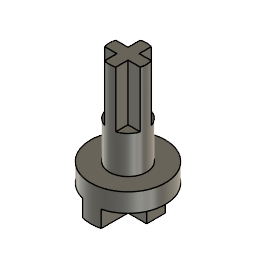
Potentiometer Axle Big (Autodesk Fusion 360 design; units mm, degrees)
part number: 2026-06-04-00-10-09-954
Autodesk Fusion 360 part; units mm, degrees
sketch "Sketch1" plane through (0, 0, 0) normal (0, 0, 1) x (1, 0, 0)
  circle A0 centre (0, 0) radius 1
  constraint coincident A0.centre origin
extrude "Extrude1" add sketch "Sketch1" along normal blind 0.5
sketch "Sketch2" plane through (0, 0, 0.5) normal (0, 0, 1) x (-1, 0, 0)
  circle A0 centre (0, 0) radius 1
  circle A1 centre (0, 0) radius 0.5
  constraint concentric A0 A1
extrude "Extrude2" add sketch "Sketch2" along normal blind 1 contours A1
sketch "Sketch3" plane through (0, 0, 1.5) normal (0, 0, 1) x (-1, 0, 0)
  circle A0 centre (0, 0) radius 0.5
  arc A1 (-0.1, -0.4899) -> (0.0992, -0.4901) centre (0, 0) ccw
  arc A2 (0.4899, -0.1) -> (0.4901, 0.0992) centre (0, 0) ccw
  arc A3 (0.1, 0.4899) -> (-0.1, 0.4899) centre (0, 0) ccw
  arc A4 (-0.4899, 0.1) -> (-0.4899, -0.1) centre (0, 0) ccw
  arc A5 (-0.15, -0.477) -> (0.15, -0.477) centre (0, 0) ccw
  arc A6 (-0.477, 0.15) -> (-0.477, -0.15) centre (0, 0) ccw
  arc A7 (0.477, -0.15) -> (0.477, 0.15) centre (0, 0) ccw
  arc A8 (0.15, 0.477) -> (-0.15, 0.477) centre (0, 0) ccw
  line L0 (-0.15, -0.15) -> (-0.15, -0.45)
  line L1 (-0.15, -0.45) -> (-0.15, -0.477)
  line L2 (-0.15, -0.15) -> (-0.477, -0.15)
  line L3 (0.15, -0.15) -> (0.15, -0.477)
  line L4 (0.15, -0.15) -> (0.477, -0.15)
  line L5 (-0.15, 0.15) -> (-0.477, 0.15)
  line L6 (-0.15, 0.15) -> (-0.15, 0.477)
  line L7 (0.15, 0.15) -> (0.15, 0.477)
  line L8 (0.15, 0.15) -> (0.477, 0.15)
  constraint concentric A0 A1
  constraint coincident A0 A3.end
  constraint concentric A1 A4
  constraint concentric A2 A3
  constraint concentric A3 A4
  constraint concentric A3 A8
  constraint concentric A5 A7
  constraint concentric A6 A8
  constraint concentric A7 A8
  constraint parallel L0 L1
  constraint coincident A0 A5.start
  constraint perpendicular L0 L2
  constraint vertical L3
  constraint perpendicular L3 L4
  constraint parallel L2 L5
  constraint perpendicular L5 L6
  constraint perpendicular L4 L7
  constraint perpendicular L7 L8
  constraint coincident A0 A8.start
extrude "Extrude4" add sketch "Sketch3" along normal blind 1 contours A0 A1 A2 A3 A4 A5 A6 A7 A8 L0 L1 L2 L3 L4 L5 L6 L7 L8
sketch "Sketch4" plane through (0, 0, 0) normal (0, 0, -1) x (1, 0, 0)
  circle A0 centre (0, 0) radius 1
  line L0 (0.25, -0.25) -> (0.25, -0.9682)
  line L1 (0.25, 0.9682) -> (0.25, 0.25)
  line L2 (0.25, 0.25) -> (0.75, 0.25)
  line L3 (0.75, 0.25) -> (0.75, -0.25)
  line L4 (-0.75, -0.25) -> (-0.75, 0.25)
  line L5 (-0.75, 0.25) -> (-0.25, 0.25)
  line L6 (-0.25, -0.9682) -> (-0.25, -0.25)
  line L7 (-0.25, 0.25) -> (-0.25, 0.9682)
  arc A1 (0.25, 0.9682) -> (-0.25, 0.9682) centre (0, 0) ccw
  arc A2 (-0.25, -0.9682) -> (0.25, -0.9682) centre (0, 0) ccw
  line L8 (0.75, -0.25) -> (0.25, -0.25)
  line L9 (-0.25, -0.25) -> (-0.75, -0.25)
  constraint coincident A0.centre A1.centre
  constraint coincident A0 L1.start
  constraint coincident A0 L7.end
  constraint coincident A0 L0.end
  constraint coincident A0 L6.start
  constraint perpendicular L1 L2
  constraint perpendicular L2 L3
  constraint perpendicular L6 L9
  constraint perpendicular L4 L9
  constraint perpendicular L5 L7
  constraint collinear L6 L7
  constraint concentric A1 A2
  constraint collinear L8 L9
extrude "Extrude5" add sketch "Sketch4" along normal blind 0.45 contours A0 L0 L1 L2 L3 L4 L5 L6 L7 A1 A2 L8 L9
extrude "Extrude6" add 1 faces at (-0.2667, 0, 2.5) along direction (0, 0, 1) blind 0.5
